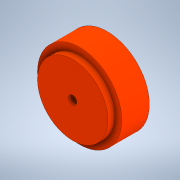
# Autodesk Inventor part: FootSensorCalibrationTool
Saved by Autodesk Inventor 2022.2 (Build 262287030, 287C)
## iProperties
Created: 2022-02-23
Part Number: FootSensorCalibrationTool
Material: Generic
Document SubType Name: Modeling
Designer: Jochen
Density: 1 g/cm^3
Appearance: Default
Author: Jochen
Autodesk Inventor part; units mm, degrees
ref_plane "YZ Plane" through (0, 0, 0) normal (1, 0, 0) x (0, 1, 0)
ref_plane "XZ Plane" through (0, 0, 0) normal (0, 1, 0) x (-1, 0, 0)
ref_plane "XY Plane" through (0, 0, 0) normal (0, 0, 1) x (1, 0, 0)
sketch "Sketch1" plane through (0, 0, 0) normal (0, 0, 1) x (1, 0, 0)
  line L0 (-8.54, 0) -> (8.54, 0) construction
  line L1 (0, -8.54) -> (0, 8.54) construction
  circle A0 centre (0, 0) radius 0.6
  circle A1 centre (0, 0) radius 5.1
  circle A2 centre (0, 0) radius 6.1
  dimension "d0" = 1.2
  dimension "d1" = 10.2
  dimension "d4" = 1
  constraints: 3 centre point, 3 coincident
  measures "d0" diameter of A0
  measures "d1" diameter of A1
  measures "d4" radial gap between concentric circles of A2 A1
extrude "Extrusion1" add sketch "Sketch1" along normal blind 1 contours A1
extrude "Extrusion2" add sketch "Sketch1" against normal blind 4 contours A1 | A2
body "Solid1"
